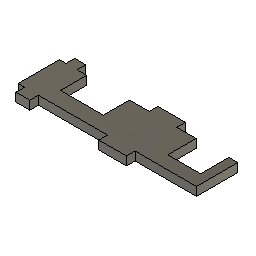
Activity1Solution v2 (Autodesk Fusion 360 design; units mm, degrees)
Autodesk Fusion 360 part; units mm, degrees
sketch "Sketch1" plane through (0, 0, 0) normal (0, 0, 1) x (1, 0, 0)
  line L0 (15, 20) -> (15, 32)
  line L1 (15, 32) -> (16.9, 32)
  line L2 (15, 20) -> (16.9, 20)
  line L3 (16.9, 32) -> (16.9, 34.5)
  line L4 (16.9, 20) -> (16.9, 17.5)
  line L5 (16.9, 34.5) -> (20.1, 34.5)
  line L6 (16.9, 17.5) -> (20.9, 17.5)
  line L7 (20.1, 34.5) -> (20.1, 32)
  line L8 (20.9, 17.5) -> (20.9, 20)
  line L9 (20.1, 32) -> (22.9, 32)
  line L10 (22.9, 32) -> (22.9, 24.4)
  line L11 (22.9, 24.4) -> (35.3, 24.4)
  line L12 (35.3, 24.4) -> (35.3, 32)
  line L13 (35.3, 32) -> (41, 32)
  line L14 (41, 32) -> (41, 34.5)
  line L15 (41, 34.5) -> (49, 34.5)
  line L16 (49, 34.5) -> (49, 32)
  line L17 (49, 32) -> (54.7, 32)
  line L18 (20.9, 20) -> (40.9, 20)
  line L19 (40.9, 20) -> (40.9, 17.5)
  line L20 (40.9, 17.5) -> (48.9, 17.5)
  line L21 (48.9, 17.5) -> (48.9, 20)
  line L22 (48.9, 20) -> (66.7, 20)
  line L23 (66.7, 20) -> (66.7, 32)
  line L24 (66.7, 32) -> (64.1, 32)
  line L25 (64.1, 32) -> (64.1, 23.8)
  line L26 (64.1, 23.8) -> (54.6, 23.8)
  line L27 (54.6, 23.8) -> (54.6, 32)
  dimension "d1" = 12
  dimension "d2" = 1.9
  dimension "d3" = 1.9
  dimension "d4" = 2.5
  dimension "d5" = 2.5
  dimension "d6" = 3.2
  dimension "d7" = 4
  dimension "d8" = 2.5
  dimension "d9" = 2.5
  dimension "d10" = 2.8
  dimension "d11" = 7.6
  dimension "d12" = 12.4
  dimension "d13" = 7.6
  dimension "d14" = 5.7
  dimension "d15" = 2.5
  dimension "d16" = 8
  dimension "d17" = 2.5
  dimension "d18" = 5.7
  dimension "d19" = 20
  dimension "d20" = 2.5
  dimension "d21" = 8
  dimension "d22" = 2.5
  dimension "d23" = 17.8
  dimension "d24" = 12
  dimension "d25" = 2.6
  dimension "d26" = 8.2
  dimension "d27" = 9.5
  constraint vertical L0
  constraint horizontal L1
  constraint horizontal L2
  constraint perpendicular L1 L3
  constraint perpendicular L2 L4
  constraint perpendicular L3 L5
  constraint perpendicular L4 L6
  constraint perpendicular L5 L7
  constraint perpendicular L6 L8
  constraint perpendicular L7 L9
  constraint perpendicular L9 L10
  constraint perpendicular L10 L11
  constraint perpendicular L11 L12
  constraint perpendicular L12 L13
  constraint perpendicular L13 L14
  constraint perpendicular L14 L15
  constraint perpendicular L15 L16
  constraint perpendicular L16 L17
  constraint perpendicular L8 L18
  constraint perpendicular L18 L19
  constraint perpendicular L19 L20
  constraint perpendicular L20 L21
  constraint perpendicular L21 L22
  constraint perpendicular L22 L23
  constraint perpendicular L23 L24
  constraint perpendicular L24 L25
  constraint perpendicular L25 L26
  constraint coincident L17 L27.end
  constraint perpendicular L17 L27
  measures "d1" distance of L0.start L0.end
  measures "d2" distance of L0.end L1.end
  measures "d3" distance of L0.start L2.end
  measures "d4" distance of L1.end L3.end
  measures "d5" distance of L2.end L4.end
  measures "d6" distance of L3.end L5.end
  measures "d7" distance of L4.end L6.end
  measures "d8" distance of L5.end L7.end
  measures "d9" distance of L6.end L8.end
  measures "d10" distance of L7.end L9.end
  measures "d11" distance of L9.end L10.end
  measures "d12" distance of L10.end L11.end
  measures "d13" distance of L11.end L12.end
  measures "d14" distance of L12.end L13.end
  measures "d15" distance of L13.end L14.end
  measures "d16" distance of L14.end L15.end
  measures "d17" distance of L15.end L16.end
  measures "d18" distance of L16.end L17.end
  measures "d19" distance of L8.end L18.end
  measures "d20" distance of L18.end L19.end
  measures "d21" distance of L19.end L20.end
  measures "d22" distance of L20.end L21.end
  measures "d23" distance of L21.end L22.end
  measures "d24" distance of L22.end L23.end
  measures "d25" distance of L23.end L24.end
  measures "d26" distance of L24.end L25.end
  measures "d27" distance of L25.end L26.end
extrude "Extrude1" add sketch "Sketch1" along normal blind 2.5
